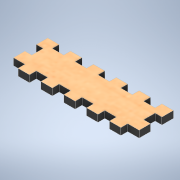
# Autodesk Inventor part: plate_front_small
Saved by Autodesk Inventor 2021 (Build 250183000, 183)
## iProperties
Created: 2021-03-07
Part Number: plate_front_small
Material: Holz (Kirsche)
Document SubType Name: Modeling
Designer: Tilman
Density: 0.63 g/cm^3
Appearance: Glänzend - Schwarz
Author: Tilman
Autodesk Inventor part; units mm, degrees
ref_plane "YZ Plane" through (0, 0, 0) normal (1, 0, 0) x (0, 1, 0)
ref_plane "XZ Plane" through (0, 0, 0) normal (0, 1, 0) x (-1, 0, 0)
ref_plane "XY Plane" through (0, 0, 0) normal (0, 0, 1) x (1, 0, 0)
sketch "Skizze1" plane through (0, 0, 0) normal (0, 1, 0) x (-1, 0, 0)
  line L0 (-5, 0) -> (-5, -3)
  line L1 (-5, -3) -> (0, -3)
  line L2 (-5, 0) -> (-10, 0)
  line L3 (-10, 0) -> (-10, -3)
  line L4 (-10, -3) -> (-15, -3)
  line L5 (-15, 0) -> (-15, -3)
  line L6 (-15, 0) -> (-20, 0)
  line L7 (-20, 0) -> (-20, -3)
  line L8 (-20, -3) -> (-25, -3)
  line L9 (-25, 0) -> (-25, -3)
  line L10 (-25, 0) -> (-30, 0)
  line L11 (-30, 0) -> (-30, -3)
  line L12 (-30, -3) -> (-35, -3)
  line L13 (-35, 0) -> (-35, -3)
  line L14 (-35, 0) -> (-40, 0)
  line L15 (-40, 0) -> (-40, -3)
  line L16 (-40, -3) -> (-45, -3)
  line L17 (-45, 0) -> (-45, -3)
  line L18 (-45, 0) -> (-50, 0)
  line L19 (-50, 0) -> (-50, -3)
  line L20 (-50, -3) -> (-55, -3)
  line L21 (-55, -3) -> (-55, -8)
  line L22 (-55, -8) -> (-52, -8)
  line L23 (-52, -8) -> (-52, -13)
  line L24 (-52, -13) -> (-55, -13)
  line L25 (0, -3) -> (0, -8)
  line L26 (0, -8) -> (-3, -8)
  line L27 (-3, -8) -> (-3, -13)
  line L28 (-3, -13) -> (0, -13)
  line L29 (0, -13) -> (0, -18)
  line L30 (-55, -18) -> (-55, -13)
  line L31 (0, -18) -> (-5, -18)
  line L32 (-5, -18) -> (-5, -15)
  line L33 (-5, -15) -> (-10, -15)
  line L34 (-10, -15) -> (-10, -18)
  line L35 (-20, -15) -> (-20, -18)
  line L36 (-15, -18) -> (-15, -15)
  line L37 (-10, -18) -> (-15, -18)
  line L38 (-15, -15) -> (-20, -15)
  line L39 (-30, -15) -> (-30, -18)
  line L40 (-25, -18) -> (-25, -15)
  line L41 (-20, -18) -> (-25, -18)
  line L42 (-25, -15) -> (-30, -15)
  line L43 (-40, -15) -> (-40, -18)
  line L44 (-35, -18) -> (-35, -15)
  line L45 (-30, -18) -> (-35, -18)
  line L46 (-35, -15) -> (-40, -15)
  line L47 (-50, -15) -> (-50, -18)
  line L48 (-45, -18) -> (-45, -15)
  line L49 (-40, -18) -> (-45, -18)
  line L50 (-45, -15) -> (-50, -15)
  line L51 (-50, -18) -> (-55, -18)
  point P0 (0, 0)
  dimension "d2" = 5
  dimension "d3" = 3
  dimension "d6" = 10
  dimension "d13" = 10
  constraints: 104 end point, 14 equal length, 12 perpendicular, 7 point on line, 5 horizontal, 4 vertical, 2 collinear, 1 horizontal alignment, 1 vertical alignment, 70 other
  measures "d2" distance of L0.start L2.end
  measures "d3" distance of L0.start L0.end
  measures "d6" distance of L0.start L5.start
  measures "d13" distance of L33.end L35.start
extrude "Extrusion1" add sketch "Skizze1" along normal blind 3
